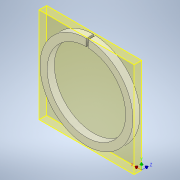
# Autodesk Inventor part: 4002_Bias_Coil_Holder_Tube_Mount_Layer2_MPSv2_v1
Saved by Autodesk Inventor 2021 (Build 250183000, 183)
## iProperties
Created: 2020-11-16
Part Number: 4002_Bias_Coil_Holder_Tube_Mount_Layer2_MPSv2_v1
Material: Acetal Resin, White
Document SubType Name: Modeling
Designer: Admin
Density: 1.425 g/cm^3
Appearance: Smooth - White
Author: Admin
Autodesk Inventor part; units mm, degrees
ref_plane "YZ Plane" through (0, 0, 0) normal (1, 0, 0) x (0, 1, 0)
ref_plane "XZ Plane" through (0, 0, 0) normal (0, 1, 0) x (-1, 0, 0)
ref_plane "XY Plane" through (0, 0, 0) normal (0, 0, 1) x (1, 0, 0)
sketch "Sketch13" plane through (0, 0, 0) normal (0, 0, 1) x (1, 0, 0)
  circle A0 centre (0, 0) radius 33
  circle A1 centre (0, 0) radius 39.038
  line L0 (0, 0) -> (0, 39.038)
  line L1 (0, 0) -> (1.7028, 39.0008)
  line L2 (0, 0) -> (39.038, 0) construction
  point P0 (1.4394, 32.9686)
  point P1 (0, 33)
  dimension "d62" = 66
  dimension "d63" = 78.076
  dimension "d64" = 87.5
  constraints: 6 end point, 2 centre point, 2 coincident, 2 point on circle, 1 equal length, 1 horizontal
  measures "d62" diameter of A0
  measures "d63" diameter of A1
  measures "d64" angle of L2 L1
extrude "Extrusion12" add sketch "Sketch13" along normal blind 6 contours A0 L1 A1 L0 picked at (-2.8956, 36.6991)
sketch "Sketch4" plane through (40, -2.75, -25.3875) normal (1, 0, 0) x (0, 0, -1)
  line L0 (-51.025, 0.25) -> (-51.6313, 0.25) projected
  line L1 (-51.025, 0.25) -> (-55.267, 0.25)
  line L2 (-55.267, 0.25) -> (-55.267, 5.25)
  line L3 (-55.267, 5.25) -> (-51.025, 5.25)
  line L4 (-51.025, 5.25) -> (-51.025, 0.25)
  point P0 (-25.3875, 2.75)
  point P1 (-51.6313, 0.25)
  dimension "d33" = 4.242
  dimension "d34" = 5
  constraints: 8 end point, 2 parallel, 1 horizontal, 1 perpendicular
  measures "d33" distance of L2.end L3.end
  measures "d34" distance of L1.end L2.end
sketch "Sketch5" plane through (40, -2.75, -25.3875) normal (1, 0, 0) x (0, 0, -1)
  line L0 (-51.6563, 0.25) -> (-55.267, 0.25) projected
  line L1 (-55.267, 5.25) -> (-51.6563, 5.25) projected
  line L2 (-55.267, 0.25) -> (-52.267, 0.25)
  line L3 (-52.267, 0.25) -> (-52.267, 5.25)
  line L4 (-52.267, 5.25) -> (-55.267, 5.25)
  line L5 (-55.267, 5.25) -> (-55.267, 0.25)
  point P0 (-25.3875, 2.75)
  point P1 (-55.267, 5.25)
  point P2 (-52.267, 0.25)
  dimension "d37" = 3
  constraints: 8 end point, 2 parallel, 1 horizontal, 1 perpendicular, 1 point on line
  measures "d37" distance of L4.end L3.end
sketch "Sketch6" plane through (220, -2.75, -25.3875) normal (1, 0, 0) x (0, 0, -1)
  line L0 (-51.6563, 0.25) -> (-55.267, 0.25) projected
  line L1 (-55.267, 0.25) -> (-51.025, 0.25)
  line L2 (-51.025, 0.25) -> (-51.025, 5.25)
  line L3 (-51.025, 5.25) -> (-55.267, 5.25)
  line L4 (-55.267, 5.25) -> (-55.267, 0.25)
  point P0 (-25.3875, 2.75)
  dimension "d40" = 4.242
  constraints: 8 end point, 2 parallel, 1 horizontal, 1 perpendicular
  measures "d40" distance of L3.end L2.end
sketch "Sketch7" plane through (30, -2.75, -25.3875) normal (-1, 0, 0) x (0, 0, 1)
  line L0 (55.267, 0.25) -> (55.267, 5.25) projected
  line L1 (55.267, 0.25) -> (58.267, 0.25)
  line L2 (58.267, 0.25) -> (58.267, 5.25)
  line L3 (58.267, 5.25) -> (55.267, 5.25)
  line L4 (55.267, 5.25) -> (55.267, 0.25)
  point P0 (25.3875, 2.75)
  dimension "d43" = 3
  dimension "d44" = 5
  constraints: 8 end point, 2 parallel, 1 horizontal, 1 perpendicular
  measures "d43" distance of L3.end L2.end
  measures "d44" distance of L2.end L1.end
sketch "Sketch8" plane through (30, -2.75, -25.3875) normal (-1, 0, 0) x (0, 0, 1)
  line L0 (51.6563, 0.25) -> (58.267, 0.25) projected
  line L1 (58.267, 5.25) -> (51.6563, 5.25) projected
  line L2 (58.267, 0.25) -> (57.025, 0.25)
  line L3 (57.025, 0.25) -> (57.025, 5.25)
  line L4 (57.025, 5.25) -> (58.267, 5.25)
  line L5 (58.267, 5.25) -> (58.267, 0.25)
  point P0 (25.3875, 2.75)
  point P1 (57.025, 0.25)
  dimension "d47" = 1.242
  constraints: 8 end point, 2 parallel, 1 horizontal, 1 perpendicular, 1 point on line
  measures "d47" distance of L3.end L4.end
sketch "Sketch9" plane through (40, -2.75, -25.3875) normal (1, 0, 0) x (0, 0, -1)
  line L0 (-52.267, 0.25) -> (-51.025, 0.25) projected
  line L1 (-51.025, 5.25) -> (-51.025, 0.25) projected
  line L2 (-52.267, 0.25) -> (-51.025, 0.25)
  line L3 (-51.025, 0.25) -> (-51.025, 5.25)
  line L4 (-51.025, 5.25) -> (-52.267, 5.25)
  line L5 (-52.267, 5.25) -> (-52.267, 0.25)
  point P0 (-25.3875, 2.75)
  constraints: 8 end point, 2 parallel, 1 horizontal, 1 perpendicular
body "Solid1"
body "Solid2"
